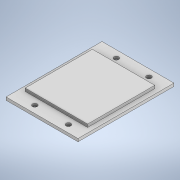
# Autodesk Inventor part: tapapic
Saved by Autodesk Inventor 2021 (Build 250183000, 183)
## iProperties
Created: 2024-01-19
Part Number: tapapic
Material: Generic
Document SubType Name: Modeling
Designer: MARCO BRAVO
Density: 1 g/cm^3
Appearance: Default
Author: MARCO BRAVO
Autodesk Inventor part; units mm, degrees
ref_plane "YZ Plane" through (0, 0, 0) normal (1, 0, 0) x (0, 1, 0)
ref_plane "XZ Plane" through (0, 0, 0) normal (0, 1, 0) x (-1, 0, 0)
ref_plane "XY Plane" through (0, 0, 0) normal (0, 0, 1) x (1, 0, 0)
sketch "Sketch1" plane through (0, 0, 0) normal (0, 1, 0) x (-1, 0, 0)
  line L0 (0, 0) -> (70, 0)
  line L1 (70, -100) -> (0, -100)
  line L2 (0, -100) -> (0, 0)
  line L3 (35, 0) -> (70, 0)
  line L4 (0, 0) -> (35, 0)
  line L5 (35, -100) -> (70, -100)
  line L6 (2.147, -100) -> (35, -100)
  circle A0 centre (52.5, -7.5) radius 2.5
  circle A1 centre (17.5, -7.5) radius 2.5
  circle A2 centre (18.5735, -92.5) radius 2.5
  circle A3 centre (52.5, -92.5) radius 2.5
  line L7 (70, -85) -> (5, -85)
  line L8 (5, -85) -> (5, -15)
  line L9 (5, -15) -> (70, -15)
  line L10 (70, -100) -> (75, -100)
  line L11 (75, -100) -> (75, 0)
  line L12 (75, 0) -> (70, 0)
  line L13 (70, -15) -> (70, -85)
  line L14 (75, 0) -> (0, 0)
  dimension "d0" = 100
  dimension "d1" = 70
  dimension "d17" = 5
  dimension "d18" = 5
  dimension "d19" = 5
  dimension "d20" = 5
  dimension "d22" = 65
  dimension "d23" = 70
  dimension "d24" = 5
  dimension "d25" = 70
  constraints: 30 end point, 4 centre point, 4 collinear, 4 perpendicular, 2 horizontal, 2 midpoint, 1 parallel, 1 point on line, 1 vertical
  measures "d0" distance of L0.end L1.start
  measures "d1" distance of L1.start L1.end
  measures "d17" diameter of A0
  measures "d18" diameter of A1
  measures "d19" diameter of A2
  measures "d20" diameter of A3
  measures "d22" distance of L7.start L7.end
  measures "d23" distance of L7.end L8.end
  measures "d24" distance of L1.start L10.end
  measures "d25" distance of L9.end L7.start
extrude "Extrusion1" add sketch "Sketch1" along normal blind 6 contours L7 L8 L9 L13
extrude "Extrusion2" add sketch "Sketch1" along normal blind 3
body "Solid1"
